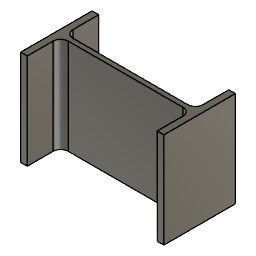
H-150×75×5×7 (Autodesk Fusion 360 design; units mm, degrees)
Autodesk Fusion 360 part; units mm, degrees
sketch "スケッチ1" plane through (0, 0, 0) normal (0, 0, 1) x (1, 0, 0)
  line L0 (0, 37.5) -> (0, -37.5)
  line L1 (150, -37.5) -> (150, 37.5)
  line L2 (143, -10.5) -> (143, -37.5)
  line L3 (7, -37.5) -> (7, -10.5)
  line L4 (0, -37.5) -> (7, -37.5)
  line L5 (143, -37.5) -> (150, -37.5)
  line L6 (135, 2.5) -> (15, 2.5)
  line L7 (15, -2.5) -> (135, -2.5)
  arc A0 (7, 10.5) -> (15, 2.5) centre (15, 10.5) ccw
  arc A1 (15, -2.5) -> (7, -10.5) centre (15, -10.5) ccw
  line L8 (7, 37.5) -> (0, 37.5)
  line L9 (7, 10.5) -> (7, 37.5)
  arc A2 (135, 2.5) -> (143, 10.5) centre (135, 10.5) ccw
  arc A3 (143, -10.5) -> (135, -2.5) centre (135, -10.5) ccw
  line L10 (143, 37.5) -> (143, 10.5)
  line L11 (150, 37.5) -> (143, 37.5)
extrude "押し出し1" add sketch "スケッチ1" along normal blind 100
